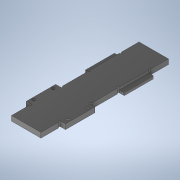
# Autodesk Inventor part: Cockpit_lower_bottom_frame
Saved by Autodesk Inventor 2020 (Build 240168000, 168)
## iProperties
Created: 2021-04-12
Part Number: Cockpit_lower_bottom_frame
Material: アセタール樹脂、黒
Document SubType Name: Modeling
Designer: Masato Kubotera
Density: 1.425 g/cm^3
Appearance: 滑らか - 黒
Mass: 18.7737 g
Surface Area: 103.06 cm^2
Volume: 13.1745 cm^3
Description: POM T5
Author: Masato Kubotera
Title: Cockpit_horizontal_frame_03
Autodesk Inventor part; units mm, degrees
ref_plane "YZ Plane" through (0, 0, 0) normal (1, 0, 0) x (0, 1, 0)
ref_plane "XZ Plane" through (0, 0, 0) normal (0, 1, 0) x (-1, 0, 0)
ref_plane "XY Plane" through (0, 0, 0) normal (0, 0, 1) x (1, 0, 0)
sketch "スケッチ1" plane through (0, 0, 0) normal (0, 0, 1) x (1, 0, 0)
  line L0 (-15, 65) -> (15, 65)
  line L1 (15, 65) -> (15, 47.1)
  line L2 (15, -65) -> (-15, -65)
  line L3 (-15, -65) -> (-15, -47.1)
  line L4 (-15, 65) -> (15, -65) construction
  line L5 (15, 65) -> (-15, -65) construction
  line L6 (-15, 45) -> (-20, 45)
  line L7 (-20, 45) -> (-20, 45)
  line L8 (-20, 15) -> (-15, 15)
  line L9 (-20, 15) -> (-20, 45)
  line L10 (-15, -15) -> (-20, -15)
  line L11 (-20, -15) -> (-20, -45)
  line L12 (-20, -45) -> (-15, -45)
  arc A0 (-15, 45) -> (-15, 47.1) centre (-15, 46.05) ccw
  arc A1 (-15, 12.9) -> (-15, 15) centre (-15, 13.95) ccw
  arc A2 (-15, -15) -> (-15, -12.9) centre (-15, -13.95) ccw
  arc A3 (-15, -47.1) -> (-15, -45) centre (-15, -46.05) ccw
  line L13 (-15, 47.1) -> (-15, 65)
  line L14 (-15, 12.9) -> (-15, 47.1) construction
  line L15 (-15, -12.9) -> (-15, 12.9)
  line L16 (-15, -47.1) -> (-15, -45) construction
  line L17 (0, 65) -> (0, -65) construction
  line L18 (15, 45) -> (20, 45)
  line L19 (20, 15) -> (15, 15)
  line L20 (20, 15) -> (20, 45)
  line L21 (15, -15) -> (20, -15)
  line L22 (20, -15) -> (20, -45)
  line L23 (20, -45) -> (15, -45)
  arc A4 (15, 47.1) -> (15, 45) centre (15, 46.05) ccw
  arc A5 (15, 15) -> (15, 12.9) centre (15, 13.95) ccw
  arc A6 (15, -12.9) -> (15, -15) centre (15, -13.95) ccw
  arc A7 (15, -45) -> (15, -47.1) centre (15, -46.05) ccw
  line L24 (15, 47.1) -> (15, 12.9) construction
  line L25 (15, 12.9) -> (15, -12.9)
  line L26 (15, -47.1) -> (15, -65)
  line L27 (15, -12.9) -> (15, -15) construction
  circle A8 centre (-17.5, 40) radius 1.55
  circle A9 centre (-17.5, 20) radius 1.55
  circle A10 centre (17.5, 20) radius 1.55
  circle A11 centre (17.5, 40) radius 1.55
  line L28 (-15, -15) -> (-15, -12.9) construction
  line L29 (-15, -45) -> (-15, -15)
  line L30 (15, -15) -> (15, -45)
  line L31 (15, -45) -> (15, -47.1) construction
  point P0 (0, 0)
  dimension "d8" = 30
  dimension "d9" = 130
  dimension "d10" = 20
  dimension "d11" = 30
  dimension "d12" = 30
  dimension "d13" = 30
  dimension "d16" = 1.05
  dimension "d17" = 1.05
  dimension "d18" = 1.05
  dimension "d19" = 1.05
  dimension "d20" = 5
  dimension "d23" = 20
  dimension "d24" = 5
  dimension "d25" = 5
  dimension "d28" = 2.5
  dimension "d29" = 2.5
  dimension "d33" = 3.1
  dimension "d38" = 3.1
  dimension "d39" = 20
  constraints: 62 end point, 43 parallel, 26 perpendicular, 18 symmetric about line, 16 point on circle, 12 centre point, 7 vertical, 6 midpoint, 5 horizontal, 5 point on line, 1 collinear, 17 other
  measures "d8" distance of L0.start L0.end
  measures "d9" distance of L0.end L2.start
  measures "d10" distance between parallel lines of L6 L0
  measures "d11" distance of L8.start L6.end
  measures "d12" distance between parallel lines of L10 L8
  measures "d13" distance of L10.end L11.end
  measures "d16" radius of A0
  measures "d17" radius of A1
  measures "d18" radius of A2
  measures "d19" radius of A3
  measures "d20" distance between parallel lines of L9 L13
  measures "d23" distance between parallel lines of L2 L12
  measures "d24" distance from line of L6 A8.centre
  measures "d25" distance from line of L8 A9.centre
  measures "d28" distance from line of L9 A8.centre
  measures "d29" distance from line of L9 A9.centre
  measures "d33" diameter of A9
  measures "d38" diameter of A8
  measures "d39" distance of A9.centre A8.centre
extrude "押し出し1" add sketch "スケッチ1" along normal blind 2.5
extrude "押し出し2" add sketch "スケッチ1" along normal blind 5 contours L0 L1 A4 L18 L20 L19 A5 L25 A6 L30 A7 L26 L2 L3 A3 L29 A2 L15 A1 L8 L9 L6 A0 L13
chamfer "面取り1" distance 0.5 angle 45 4 edges at (20, -15, 1.25) (20, -45, 1.25) (-20, -15, 1.25) (-20, -45, 1.25)
equation "\"d10\" = -0.5 * d12 + 0.5 * d9 - d11"
equation "\"d13\" = d11"
equation "\"d17\" = d16"
equation "\"d18\" = d17"
equation "\"d19\" = d18"
equation "\"d25\" = d24"
equation "\"d28\" = 0.5 * d20"
equation "\"d29\" = d28"
equation "\"d33\" = d38"
